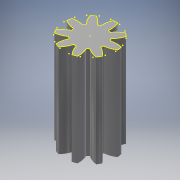
# Autodesk Inventor part: 平歯車1
Saved by Autodesk Inventor 2018.3 (Build 223284000, 284)
## iProperties
Created: 2019-04-14
Part Number: 平歯車1
Material: Steel
Document SubType Name: Modeling
Designer: shun2
Categories: <?xml version="1.0" encoding="UTF-16"?> <MemberInstance><Categories><FamilyTemplate><FamilyTemplateParameter ValueType="xs:double" Id="1" ObjectReferenceKey="da_z" ObjectType="kUserParameterObject"/><FamilyTemplateParameter ValueType="xs:double" Id="2" ObjectReferenceKey="da_b" ObjectType="kUserParameterObject"/><FamilyTemplateParameter ValueType="xs:double" Id="3" ObjectReferenceKey="da_beta" ObjectType="kUserParameterObject"/><FamilyTemplateParameter ValueType="xs:double" Id="4" ObjectReferenceKey="da_da" ObjectType="kUserParameterObject"/><FamilyTemplateParameter ValueType="xs:double" Id="5" ObjectReferenceKey="da_aw" ObjectType="kUserParameterObject"/><FamilyTemplateParameter ValueType="xs:string" Id="6" ObjectReferenceKey="EAIAABAAAACIAQAAAAAAAIAAAAAAAAAA" ObjectType="83910656" SubObjectId="SurfaceGeometry"/></FamilyTemplate><ParamToTemplateMap><ParamToTemplate CategoryParameter="//CategoryParameter[@InternalName='046C89C9-8512-4d59-83FE-43B91F4F132A']" TemplateParameter="1"/><ParamToTemplate CategoryParameter="//CategoryParameter[@InternalName='2552DF32-E462-4b46-AEBF-C6C7768E72AC']" TemplateParameter="2"/><ParamToTemplate CategoryParameter="//CategoryParameter[@InternalName='C9EE641D-15FC-4fae-A226-E94C4372FDD7']" TemplateParameter="3"/><ParamToTemplate><ParamToTemplate CategoryParameter="//CategoryParameter[@InternalName='00B6519A-459B-49c7-AD84-2E56D39A5744']" ConstantValue="0.000000"/></ParamToTemplate><ParamToTemplate><ParamToTemplate CategoryParameter="//CategoryParameter[@InternalName='04B31F0E-C7A6-4894-AA32-9629BEFACF47']" ConstantValue="1.000000"/></ParamToTemplate><ParamToTemplate><ParamToTemplate CategoryParameter="//CategoryParameter[@InternalName='43CBEC2E-7847-49e7-A936-2F7889FCB2D9']" ConstantValue="0.250000"/></ParamToTemplate><ParamToTemplate><ParamToTemplate CategoryParameter="//CategoryParameter[@InternalName='B1EFC894-105D-4ebd-86BF-FA20ED196853']" ConstantValue="0.333500"/></ParamToTemplate><ParamToTemplate><ParamToTemplate CategoryParameter="//CategoryParameter[@InternalName='51175063-3D10-4879-93E8-6246FE8B403D']" ConstantValue="2060000000.000000"/></ParamToTemplate><ParamToTemplate><ParamToTemplate CategoryParameter="//CategoryParameter[@InternalName='A3A52E27-4454-46a9-B0BD-C932399B70AF']" ConstantValue="0.300000"/></ParamToTemplate><ParamToTemplate><ParamToTemplate CategoryParameter="//CategoryParameter[@InternalName='91B76062-C214-41d9-B1B9-14D2AB99603D']" ConstantValue="0.100000"/></ParamToTemplate><ParamToTemplate><ParamToTemplate CategoryParameter="//CategoryParameter[@InternalName='374E806E-8B8A-4dda-A9AA-1039D6500AD2']" ConstantValue="10.000000"/></ParamToTemplate><ParamToTemplate><ParamToTemplate CategoryParameter="//CategoryParameter[@InternalName='2D373A89-B862-43d6-8D0B-0CBF12AB9F6C']" ConstantValue="0.523599"/></ParamToTemplate><ParamToTemplate CategoryParameter="//CategoryParameter[@InternalName='37777632-D6A2-4fac-9D53-DB8ACD95C989']" TemplateParameter="4"/><ParamToTemplate CategoryParameter="//CategoryParameter[@InternalName='FD1017F1-B727-4f7e-9707-0F86F1FF9423']" TemplateParameter="5"/><ParamToTemplate><ParamToTemplate CategoryParameter="//CategoryParameter[@InternalName='9E1B4470-B2D3-4ff1-B813-535BB4CDF51A']" ConstantValue="3520000.000000"/></ParamToTemplate><ParamToTemplate><ParamToTemplate CategoryParameter="//CategoryParameter[@InternalName='F8452263-BFF6-458c-9FB1-07C4B99E95CD']" ConstantValue="11400000.000000"/></ParamToTemplate><ParamToTemplate><ParamToTemplate CategoryParameter="//CategoryParameter[@InternalName='3E3BB259-FD49-497f-8171-6EBC954A3479']" ConstantValue="2.000000"/></ParamToTemplate><ParamToTemplate CategoryParameter="//CategoryParameter[@InternalName='27C3BAF2-7550-4e4b-AE2C-0DB134B7D9B7']" TemplateParameter="6"/></ParamToTemplateMap><Category DisplayName="Gear" InternalName="DC85795E-93AB-48d5-8EEE-5A27447B64BD" Mnemonic="Gear"><CategoryParameter DisplayName="z" InternalName="046C89C9-8512-4d59-83FE-43B91F4F132A" Mnemonic="z"/><CategoryParameter DisplayName="b" InternalName="2552DF32-E462-4b46-AEBF-C6C7768E72AC" Mnemonic="b"/><CategoryParameter DisplayName="||b|" InternalName="C9EE641D-15FC-4fae-A226-E94C4372FDD7" Mnemonic="beta"/><CategoryParameter DisplayName="x" InternalName="00B6519A-459B-49c7-AD84-2E56D39A5744" Mnemonic="x"/><CategoryParameter DisplayName="a*" InternalName="04B31F0E-C7A6-4894-AA32-9629BEFACF47" Mnemonic="a"/><CategoryParameter DisplayName="c*" InternalName="43CBEC2E-7847-49e7-A936-2F7889FCB2D9" Mnemonic="c"/><CategoryParameter DisplayName="r|.f|*" InternalName="B1EFC894-105D-4ebd-86BF-FA20ED196853" Mnemonic="rf"/><CategoryParameter DisplayName="E" InternalName="51175063-3D10-4879-93E8-6246FE8B403D" Mnemonic="E"/><CategoryParameter DisplayName="||m|" InternalName="A3A52E27-4454-46a9-B0BD-C932399B70AF" Mnemonic="mi"/><Category DisplayName="SpurGear" InternalName="26C5A22E-A91E-4dfd-A3B3-23CCAFAE1764" Mnemonic="SpurGear"><CategoryParameter DisplayName="m" InternalName="91B76062-C214-41d9-B1B9-14D2AB99603D" Mnemonic="m"/><CategoryParameter DisplayName="P" InternalName="374E806E-8B8A-4dda-A9AA-1039D6500AD2" Mnemonic="PP"/><CategoryParameter DisplayName="||a|" InternalName="2D373A89-B862-43d6-8D0B-0CBF12AB9F6C" Mnemonic="alpha"/><CategoryParameter DisplayName="d|.a|" InternalName="37777632-D6A2-4fac-9D53-DB8ACD95C989" Mnemonic="da"/><CategoryParameter DisplayName="a|.w|" InternalName="FD1017F1-B727-4f7e-9707-0F86F1FF9423" Mnemonic="aw"/><CategoryParameter DisplayName="||s||.Flim|" InternalName="9E1B4470-B2D3-4ff1-B813-535BB4CDF51A" Mnemonic="sFlim"/><CategoryParameter DisplayName="||s||.Hlim|" InternalName="F8452263-BFF6-458c-9FB1-07C4B99E95CD" Mnemonic="sHlim"/><CategoryParameter DisplayName="種類" InternalName="3E3BB259-FD49-497f-8171-6EBC954A3479" Mnemonic="type"/><CategoryParameter DisplayName="PitchDiameter" InternalName="27C3BAF2-7550-4e4b-AE2C-0DB134B7D9B7" Mnemonic="IDS_PITCHDIAM"/></Category></Category></Categories></MemberInstance>
Density: 1 g/cm^3
Appearance: Steel
CustomPartVersion: 1
Author: shun2
Autodesk Inventor part; units mm, degrees
sketch "Sketch1" plane through (0, 0, 0) normal (0, 0, 1) x (1, 0, 0)
  circle A0 centre (0, 0) radius 5.5
  dimension "d0" = 11
  constraints: 1 centre point
  measures "d0" diameter of A0
extrude "Extrusion1" add sketch "Sketch1" along normal blind 20
ref_plane "Work Plane2" through (0, 0, 10) normal (0, 0, 1) x (1, 0, 0)
sketch "Sketch2" plane through (0, 0, 0) normal (0, 0, -1) x (-1, 0, 0)
  circle A0 centre (0, 0) radius 5.5 projected
  circle A1 centre (0, 0) radius 4.5
  dimension "d3" = 9
  constraints: 1 centre point, 1 coincident
  measures "d3" diameter of A1
surface extrude "ピッチ円直径" sketch "Sketch2" against normal through all shown no curves A1
ref_plane "Work Plane8" through (0, 0, 0) normal (0.9396926, 0.3420201, 0) x (0, 0, 1)
ref_plane "Work Plane9" through (0, 0, 0) normal (1, 0, 0) x (0, 1, 0)
spur gear teeth "平歯車" teeth 9 pitch diameter 9 tip diameter 11 root diameter 6.5 face width 20 start plane through (0, 0, 0) normal (0, 0, -1) x (-1, 0, 0)
sketch "スケッチ3" plane through (0, 0, 20) normal (0, 0, 1) x (1, 0, 0)
  arc A0 (-3.8891, 3.8891) -> (-2.6622, 1.8641) centre (0.9613, 5.4436) ccw projected
  arc A1 (-2.6622, 1.8641) -> (-2.9455, 1.3735) centre (0, 0) ccw projected
  arc A2 (-2.9455, 1.3735) -> (-5.3126, 1.4235) centre (-4.2337, -3.5543) ccw projected
  arc A3 (-5.3126, 1.4235) -> (-5.4791, 0.4794) centre (0, 0) ccw projected
  arc A4 (-5.4791, 0.4794) -> (-3.2376, -0.2833) centre (-2.7627, 4.7879) ccw projected
  arc A5 (-3.2376, -0.2833) -> (-3.1393, -0.8412) centre (0, 0) ccw projected
  arc A6 (-3.1393, -0.8412) -> (-4.9847, -2.3244) centre (-0.9585, -5.4441) ccw projected
  arc A7 (-4.9847, -2.3244) -> (-4.5053, -3.1547) centre (0, 0) ccw projected
  arc A8 (-4.5053, -3.1547) -> (-2.2981, -2.2981) centre (-5.194, 1.8919) ccw projected
  arc A9 (-2.2981, -2.2981) -> (-1.8641, -2.6622) centre (0, 0) ccw projected
  arc A10 (-1.8641, -2.6622) -> (-2.3244, -4.9847) centre (2.7651, -4.7865) ccw projected
  arc A11 (-2.3244, -4.9847) -> (-1.4235, -5.3126) centre (0, 0) ccw projected
  arc A12 (-1.4235, -5.3126) -> (-0.2833, -3.2376) centre (-5.1949, -1.8893) ccw projected
  arc A13 (-0.2833, -3.2376) -> (0.2833, -3.2376) centre (0, 0) ccw projected
  arc A14 (0.2833, -3.2376) -> (1.4235, -5.3126) centre (5.1949, -1.8893) ccw projected
  arc A15 (1.4235, -5.3126) -> (2.3244, -4.9847) centre (0, 0) ccw projected
  arc A16 (2.3244, -4.9847) -> (1.8641, -2.6622) centre (-2.7651, -4.7865) ccw projected
  arc A17 (1.8641, -2.6622) -> (2.2981, -2.2981) centre (0, 0) ccw projected
  arc A18 (2.2981, -2.2981) -> (4.5053, -3.1547) centre (5.194, 1.8919) ccw projected
  arc A19 (4.5053, -3.1547) -> (4.9847, -2.3244) centre (0, 0) ccw projected
  arc A20 (4.9847, -2.3244) -> (3.1393, -0.8412) centre (0.9585, -5.4441) ccw projected
  arc A21 (3.1393, -0.8412) -> (3.2376, -0.2833) centre (0, 0) ccw projected
  arc A22 (3.2376, -0.2833) -> (5.4791, 0.4794) centre (2.7627, 4.7879) ccw projected
  arc A23 (5.4791, 0.4794) -> (5.3126, 1.4235) centre (0, 0) ccw projected
  arc A24 (5.3126, 1.4235) -> (2.9455, 1.3735) centre (4.2337, -3.5543) ccw projected
  arc A25 (2.9455, 1.3735) -> (2.6622, 1.8641) centre (0, 0) ccw projected
  arc A26 (2.6622, 1.8641) -> (3.8891, 3.8891) centre (-0.9613, 5.4436) ccw projected
  arc A27 (3.8891, 3.8891) -> (3.1547, 4.5053) centre (0, 0) ccw projected
  arc A28 (3.1547, 4.5053) -> (1.3735, 2.9455) centre (5.5278, -0.0014) ccw projected
  arc A29 (1.3735, 2.9455) -> (0.8412, 3.1393) centre (0, 0) ccw projected
  arc A30 (0.8412, 3.1393) -> (0.4794, 5.4791) centre (-4.2354, 3.5521) ccw projected
  arc A31 (0.4794, 5.4791) -> (-0.4794, 5.4791) centre (0, 0) ccw projected
  arc A32 (-0.4794, 5.4791) -> (-0.8412, 3.1393) centre (4.2354, 3.5521) ccw projected
  arc A33 (-0.8412, 3.1393) -> (-1.3735, 2.9455) centre (0, 0) ccw projected
  arc A34 (-1.3735, 2.9455) -> (-3.1547, 4.5053) centre (-5.5278, -0.0014) ccw projected
  arc A35 (-3.1547, 4.5053) -> (-3.8891, 3.8891) centre (0, 0) ccw projected
equation "\"d0\" = da_da"
equation "\"d1\" = da_b"
equation "\"d3\" = da_dw"
equation "\"da_da\" = 11"
equation "\"da_b\" = 20"
equation "\"da_dw\" = 9"
body "Solid1"
body "Srf1"
